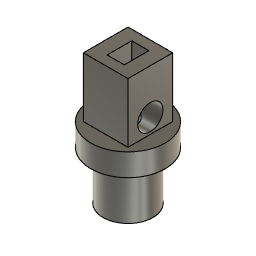
Single_Protected_Pin (Autodesk Fusion 360 design; units mm, degrees)
Autodesk Fusion 360 part; units mm, degrees
sketch "Sketch1" plane through (0, 0, 0) normal (0, 0, 1) x (1, 0, 0)
  circle A0 centre (0, 0) radius 3.35
  circle A1 centre (0, 0) radius 1.25
  dimension "d1" = 6.7
  dimension "d2" = 2.5
  constraint coincident A0.centre A1.centre
  constraint concentric A0 A1
  measures "d1" diameter of A0
  measures "d2" diameter of A1
extrude "Extrude1" add sketch "Sketch1" along normal blind 6
sketch "Sketch2" plane through (0, 0, 6) normal (0, 0, 1) x (-1, 0, 0)
  circle A0 centre (0, 0) radius 1.25
  circle A1 centre (0, 0) radius 3.35
  circle A2 centre (0, 0) radius 5
  dimension "d5" = 10
  constraint coincident A0.centre A1.centre
  measures "d5" diameter of A2
extrude "Extrude2" add sketch "Sketch2" along normal blind 3 contours A1 | A2
sketch "Sketch3" plane through (0, 0, 9) normal (0, 0, 1) x (-1, 0, 0)
  circle A0 centre (0, 0) radius 1.25
  circle A1 centre (0, 0) radius 5
  line L0 (0, 0) -> (0, -3)
  line L1 (0, -3) -> (-3, -3)
  line L2 (-3, -3) -> (-3, 0)
  line L3 (-3, 0) -> (-3, 3)
  line L4 (-3, 3) -> (0, 3)
  line L5 (0, 3) -> (3, 3)
  line L6 (3, 3) -> (3, -3)
  line L7 (3, -3) -> (0, -3)
  constraint coincident A0.centre A1.centre
  constraint vertical L0
  constraint perpendicular L0 L1
  constraint perpendicular L1 L2
  constraint parallel L2 L3
  constraint perpendicular L2 L4
  constraint perpendicular L2 L5
  constraint perpendicular L5 L6
  constraint perpendicular L0 L7
extrude "Extrude3" add sketch "Sketch3" along normal blind 4 contours L1 L2 L3 L4 L5 L6 L7
sketch "Sketch4" plane through (3, 0, 0) normal (1, 0, 0) x (0, 1, 0)
  line L0 (-3, 9) -> (3, 9)
  line L1 (3, 9) -> (3, 13)
  line L2 (3, 13) -> (-3, 13)
  line L3 (-3, 13) -> (-3, 9)
  circle A0 centre (0, 11.0197) radius 1.7
  dimension "d11" = 3.4
  measures "d11" diameter of A0
extrude "Extrude4" cut sketch "Sketch4" against normal blind 3 contours A0
sketch "Sketch6" plane through (0, 0, 13) normal (0, 0, 1) x (-1, 0, 0)
  circle A0 centre (0, 0) radius 1.25
  line L0 (3, -3) -> (3, 3)
  line L1 (3, 3) -> (-3, 3)
  line L2 (-3, 3) -> (-3, -3)
  line L3 (-3, -3) -> (3, -3)
  circle A1 centre (0, 0) radius 1.2
  constraint coincident A0.centre A1.centre
extrude "Extrude5" add sketch "Sketch6" along normal blind 4 contours A0 | L0 L1 L2 L3 | A1
sketch "Sketch7" plane through (0, 0, 17) normal (0, 0, 1) x (-1, 0, 0)
  line L0 (-3, -3) -> (3, -3)
  line L1 (3, -3) -> (3, 3)
  line L2 (3, 3) -> (-3, 3)
  line L3 (-3, 3) -> (-3, -3)
  line L4 (-1.15, 0) -> (-1.15, 1.65)
  line L5 (-1.15, 0) -> (-1.15, -1.65)
  line L6 (-1.15, -1.65) -> (1.15, -1.65)
  line L7 (-1.15, 1.65) -> (1.15, 1.65)
  line L8 (1.15, 1.65) -> (1.15, -1.65)
  dimension "d20" = 2.3
  dimension "d21" = 3.3
  constraint perpendicular L5 L6
  constraint perpendicular L4 L7
  constraint perpendicular L6 L8
  measures "d20" distance of L5.end L6.end
  measures "d21" distance of L6 L7
extrude "Extrude6" cut sketch "Sketch7" against normal blind 2.5 contours L4 L5 L6 L7 L8
extrude "Extrude7" add 1 faces at (1.9625, -1.7625, 0) along direction (0, 0, -1) blind 0.5
